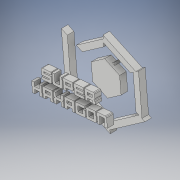
# Autodesk Inventor part: Super-Haxagon
Saved by Autodesk Inventor 2017 (Build 210142000, 142)
## iProperties
Created: 2016-12-10
Part Number: Super-Haxagon
Material: Generic
Document SubType Name: Modeling
Designer: AJ
Density: 1 g/cm^3
Appearance: Default
Author: AJ
Autodesk Inventor part; units mm, degrees
ref_plane "YZ Plane" through (0, 0, 0) normal (1, 0, 0) x (0, 1, 0)
ref_plane "XZ Plane" through (0, 0, 0) normal (0, 1, 0) x (-1, 0, 0)
sketch "Shapes" plane through (0, 0, 0) normal (0, 0, 1) x (1, 0, 0)
  circle A0 centre (0, 0) radius 63.5 construction
  line L0 (52.0162, 36.4221) -> (-5.5344, 63.2584)
  line L1 (-5.5344, 63.2584) -> (-57.5505, 26.8363)
  line L2 (-57.5505, 26.8363) -> (-52.0162, -36.4221)
  line L3 (52.0162, 36.4221) -> (57.5505, -26.8363)
  line L4 (57.5505, -26.8363) -> (5.5344, -63.2584)
  line L5 (5.5344, -63.2584) -> (-52.0162, -36.4221)
  line L6 (0, 0) -> (52.0162, 36.4221) construction
  line L7 (0, 0) -> (63.5, 0) construction
  line L8 (23.2409, 49.8402) -> (26.8363, 57.5505) construction
  line L9 (26.8363, 57.5505) -> (28.9832, 62.1546) construction
  line L10 (28.9832, 62.1546) -> (24.3791, 64.3015)
  line L11 (24.3791, 64.3015) -> (33.277, 71.3627)
  line L12 (33.277, 71.3627) -> (33.5872, 60.0077)
  line L13 (33.5872, 60.0077) -> (28.9832, 62.1546)
  line L14 (28.9832, 62.1546) -> (33.277, 71.3627) construction
  line L15 (0, 0) -> (-57.5505, 26.8363) construction
  line L16 (0, 0) -> (-52.0162, -36.4221) construction
  line L17 (0, 0) -> (5.5344, -63.2584) construction
  line L18 (0, 0) -> (57.5505, -26.8363) construction
  line L19 (0, 0) -> (-5.5344, 63.2584) construction
  line L20 (52.0162, 36.4221) -> (83.2258, 58.2754) construction
  line L21 (57.5505, -26.8363) -> (92.0809, -42.938) construction
  line L22 (5.5344, -63.2584) -> (8.855, -101.2134) construction
  line L23 (-52.0162, -36.4221) -> (-83.2258, -58.2754) construction
  line L24 (-57.5505, 26.8363) -> (-92.0809, 42.938) construction
  line L25 (-9.9619, 113.8651) -> (93.6291, 65.5598)
  line L26 (114.4355, 80.1286) -> (-12.1757, 139.1684)
  line L27 (104.0323, 72.8442) -> (115.1011, -53.6725)
  line L28 (124.8388, 87.413) -> (138.1213, -64.407)
  line L29 (126.6112, -59.0398) -> (12.1757, -139.1684)
  line L30 (149.6314, -69.7743) -> (14.3894, -164.4717)
  line L31 (13.2825, -151.8201) -> (-124.8388, -87.413)
  line L32 (15.4963, -177.1234) -> (-145.6452, -101.9819)
  line L33 (-135.242, -94.6975) -> (-149.6314, 69.7743)
  line L34 (-172.6516, 80.5088) -> (-156.0485, -109.2663)
  line L35 (-92.0809, 42.938) -> (-8.855, 101.2134)
  line L36 (-11.0688, 126.5167) -> (-115.1011, 53.6725)
  line L37 (93.6291, 65.5598) -> (114.4355, 80.1286)
  line L38 (104.0323, 72.8442) -> (124.8388, 87.413)
  line L39 (115.1011, -53.6725) -> (138.1213, -64.407)
  line L40 (126.6112, -59.0398) -> (149.6314, -69.7743)
  line L41 (12.1757, -139.1684) -> (14.3894, -164.4717)
  line L42 (13.2825, -151.8201) -> (15.4963, -177.1234)
  line L43 (-156.0485, -109.2663) -> (-135.242, -94.6975)
  line L44 (-145.6452, -101.9819) -> (-124.8388, -87.413)
  line L45 (-92.0809, 42.938) -> (-115.1011, 53.6725)
  line L46 (-8.855, 101.2134) -> (-11.0688, 126.5167)
  line L47 (-172.6516, 80.5088) -> (-149.6314, 69.7743)
  line L48 (-5.5344, 63.2584) -> (-8.855, 101.2134) construction
  line L49 (-9.9619, 113.8651) -> (-12.1757, 139.1684)
  line L50 (-8.855, 101.2134) -> (-9.9619, 113.8651)
  line L51 (93.6291, 65.5598) -> (104.0323, 72.8442)
  line L52 (115.1011, -53.6725) -> (126.6112, -59.0398)
  line L53 (-124.8388, -87.413) -> (-135.242, -94.6975)
  line L54 (12.1757, -139.1684) -> (13.2825, -151.8201)
  dimension "d0" = 127
  dimension "d1" = 35
  dimension "d2" = 5.08
  dimension "d3" = 10.16
  dimension "d4" = 5.08
  dimension "d28" = 38.1
  dimension "d29" = 25.4
  dimension "d30" = 12.7
  dimension "d31" = 12.7
  dimension "d32" = 12.7
  dimension "d33" = 12.7
  dimension "d34" = 12.7
  constraints: 110 end point, 21 collinear, 19 point on line, 16 equal length, 13 parallel, 3 perpendicular, 1 coincident, 1 horizontal, 1 midpoint, 12 other
  measures "d1" angle of L6 L7
  measures "d2" distance of L8.end L9.end
  measures "d3" distance of L9.end L11.end
  measures "d4" distance of L9.end L10.end
  measures "d28" distance of L0.end L48.end
  measures "d29" distance of L35.end L36.start
  measures "d30" distance of L48.end L25.start
  measures "d31" distance of L25.end L27.start
  measures "d32" distance of L27.end L29.start
  measures "d33" distance of L29.end L31.start
  measures "d34" distance of L31.end L33.start
extrude "Hexagon" add sketch "Shapes" along normal blind 25.4
sketch "Lift" plane through (124.8388, 87.413, 25.4) normal (0.9962, 0.0872, 0) x (0, 0, -1)
  line L0 (25.4, 0) -> (0, 0) projected
  line L1 (0, 0) -> (-101.6, 0)
  dimension "d39" = 101.6
  constraints: 2 end point, 1 horizontal
  measures "d39" distance of L0.end L1.end
ref_plane "Offset Face" through (124.8388, 87.413, 127) normal (0, 0, 1) x (1, 0, 0)
sketch "Words" plane through (124.8388, 87.413, 127) normal (0, 0, 1) x (1, 0, 0)
  line L0 (-308.6212, -54.5376) -> (20.3223, -25.7588) construction
  line L1 (20.3223, -25.7588) -> (28.8231, -122.9237) construction
  line L2 (28.8231, -122.9237) -> (-300.1204, -151.7025) construction
  line L3 (-300.1204, -151.7025) -> (-308.6212, -54.5376) construction
  line L4 (-300.1204, -151.7025) -> (-284.9384, -150.3742)
  line L5 (28.8231, -122.9237) -> (10.8917, -124.4925)
  line L6 (-297.4904, -6.9043) -> (-280.8872, -196.6794) projected
  line L7 (13.2825, -151.8201) -> (0, 0) projected
  line L8 (-72.8226, -50.9909) -> (-130.3732, -24.1547) projected
  line L9 (-129.0892, -38.8306) -> (-130.3732, -24.1547)
  line L10 (-176.8549, -123.8352) -> (-119.3044, -150.6714) projected
  line L11 (-120.5884, -135.9955) -> (-119.3044, -150.6714)
  line L12 (-245.3905, -87.2512) -> (-246.2217, -77.7509)
  line L13 (-246.2217, -77.7509) -> (-217.7439, -75.2594)
  line L14 (-217.7439, -75.2594) -> (-218.1574, -70.5324)
  line L15 (-218.1574, -70.5324) -> (-246.6353, -73.0239)
  line L16 (-246.6353, -73.0239) -> (-248.2956, -54.0464)
  spline S0 degree 2 poles (-248.2956, -54.0464) (-248.4679, -52.0768) (-247.2204, -50.5901) knots 0 0 0 1 1 1
  spline S1 degree 2 poles (-247.2204, -50.5901) (-245.9306, -49.0529) (-243.961, -48.8806) knots 0 0 0 1 1 1
  line L17 (-243.961, -48.8806) -> (-210.7561, -45.9756)
  line L18 (-210.7561, -45.9756) -> (-209.927, -55.4527)
  line L19 (-209.927, -55.4527) -> (-238.3817, -57.9422)
  line L20 (-238.3817, -57.9422) -> (-237.9661, -62.6924)
  line L21 (-237.9661, -62.6924) -> (-209.5114, -60.2029)
  line L22 (-209.5114, -60.2029) -> (-207.8511, -79.1804)
  spline S2 degree 2 poles (-207.8511, -79.1804) (-207.6747, -81.1963) (-208.9686, -82.6871) knots 0 0 0 1 1 1
  spline S3 degree 2 poles (-208.9686, -82.6871) (-210.2624, -84.1779) (-212.1857, -84.3462) knots 0 0 0 1 1 1
  line L23 (-212.1857, -84.3462) -> (-245.3905, -87.2512)
  spline S4 degree 2 poles (-198.8157, -83.1764) (-200.8316, -83.3528) (-202.3183, -82.1053) knots 0 0 0 1 1 1
  spline S5 degree 2 poles (-202.3183, -82.1053) (-203.8091, -80.8114) (-203.9815, -78.8419) knots 0 0 0 1 1 1
  line L24 (-203.9815, -78.8419) -> (-206.8865, -45.637)
  line L25 (-206.8865, -45.637) -> (-197.3862, -44.8058)
  line L26 (-197.3862, -44.8058) -> (-194.8967, -73.2605)
  line L27 (-194.8967, -73.2605) -> (-175.9192, -71.6002)
  line L28 (-175.9192, -71.6002) -> (-178.4086, -43.1455)
  line L29 (-178.4086, -43.1455) -> (-168.9315, -42.3164)
  line L30 (-168.9315, -42.3164) -> (-165.6108, -80.2714)
  line L31 (-165.6108, -80.2714) -> (-198.8157, -83.1764)
  line L32 (-161.7412, -79.9328) -> (-165.0618, -41.9778)
  line L33 (-165.0618, -41.9778) -> (-127.1068, -38.6572)
  line L34 (-127.1068, -38.6572) -> (-125.0309, -62.3849)
  spline S6 degree 2 poles (-125.0309, -62.3849) (-124.8566, -64.3776) (-126.1504, -65.8684) knots 0 0 0 1 1 1
  spline S7 degree 2 poles (-126.1504, -65.8684) (-127.4443, -67.3592) (-129.3675, -67.5275) knots 0 0 0 1 1 1
  line L35 (-129.3675, -67.5275) -> (-153.072, -69.6013)
  line L36 (-153.072, -69.6013) -> (-152.2409, -79.1017)
  line L37 (-152.2409, -79.1017) -> (-161.7412, -79.9328)
  line L38 (-134.9237, -58.4638) -> (-135.7548, -48.9635)
  line L39 (-135.7548, -48.9635) -> (-154.7323, -50.6238)
  line L40 (-154.7323, -50.6238) -> (-153.9012, -60.1242)
  line L41 (-153.9012, -60.1242) -> (-134.9237, -58.4638)
  spline S8 degree 2 poles (-115.1664, -75.8581) (-117.1823, -76.0344) (-118.669, -74.7869) knots 0 0 0 1 1 1
  spline S9 degree 2 poles (-118.669, -74.7869) (-120.1598, -73.4931) (-120.3321, -71.5235) knots 0 0 0 1 1 1
  line L42 (-120.3321, -71.5235) -> (-123.2372, -38.3186)
  line L43 (-123.2372, -38.3186) -> (-85.2821, -34.998)
  line L44 (-85.2821, -34.998) -> (-84.453, -44.4752)
  line L45 (-84.453, -44.4752) -> (-112.9077, -46.9646)
  line L46 (-112.9077, -46.9646) -> (-112.4921, -51.7148)
  line L47 (-112.4921, -51.7148) -> (-84.0374, -49.2253)
  line L48 (-84.0374, -49.2253) -> (-83.2062, -58.7257)
  line L49 (-83.2062, -58.7257) -> (-111.6609, -61.2151)
  line L50 (-111.6609, -61.2151) -> (-111.2474, -65.9421)
  line L51 (-111.2474, -65.9421) -> (-82.7927, -63.4527)
  line L52 (-82.7927, -63.4527) -> (-81.9615, -72.953)
  line L53 (-81.9615, -72.953) -> (-115.1664, -75.8581)
  line L54 (-78.0919, -72.6145) -> (-81.4125, -34.6595)
  line L55 (-81.4125, -34.6595) -> (-48.2076, -31.7544)
  spline S10 degree 2 poles (-48.2076, -31.7544) (-46.2381, -31.5821) (-44.7473, -32.8759) knots 0 0 0 1 1 1
  spline S11 degree 2 poles (-44.7473, -32.8759) (-43.2102, -34.1658) (-43.0419, -36.089) knots 0 0 0 1 1 1
  line L56 (-43.0419, -36.089) -> (-41.7972, -50.3163)
  spline S12 degree 2 poles (-41.7972, -50.3163) (-41.6228, -52.3091) (-42.9146, -53.823) knots 0 0 0 1 1 1
  spline S13 degree 2 poles (-42.9146, -53.823) (-44.2085, -55.3138) (-46.1317, -55.4821) knots 0 0 0 1 1 1
  spline S14 degree 2 poles (-46.1317, -55.4821) (-44.1622, -55.3098) (-42.6714, -56.6036) knots 0 0 0 1 1 1
  spline S15 degree 2 poles (-42.6714, -56.6036) (-41.1363, -57.8703) (-40.968, -59.7935) knots 0 0 0 1 1 1
  line L57 (-40.968, -59.7935) -> (-40.1368, -69.2938)
  line L58 (-40.1368, -69.2938) -> (-49.614, -70.123)
  line L59 (-49.614, -70.123) -> (-50.4452, -60.6226)
  line L60 (-50.4452, -60.6226) -> (-69.4227, -62.283)
  line L61 (-69.4227, -62.283) -> (-68.5915, -71.7833)
  line L62 (-68.5915, -71.7833) -> (-78.0919, -72.6145)
  line L63 (-51.2743, -51.1455) -> (-52.1055, -41.6451)
  line L64 (-52.1055, -41.6451) -> (-71.083, -43.3055)
  line L65 (-71.083, -43.3055) -> (-70.2518, -52.8058)
  line L66 (-70.2518, -52.8058) -> (-51.2743, -51.1455)
  line L67 (-282.0424, -150.036) -> (-285.363, -112.081)
  line L68 (-285.363, -112.081) -> (-275.8627, -111.2498)
  line L69 (-275.8627, -111.2498) -> (-274.6179, -125.4771)
  line L70 (-274.6179, -125.4771) -> (-255.6404, -123.8168)
  line L71 (-255.6404, -123.8168) -> (-256.8852, -109.5895)
  line L72 (-256.8852, -109.5895) -> (-247.408, -108.7603)
  line L73 (-247.408, -108.7603) -> (-244.0874, -146.7154)
  line L74 (-244.0874, -146.7154) -> (-253.5645, -147.5445)
  line L75 (-253.5645, -147.5445) -> (-254.8093, -133.3172)
  line L76 (-254.8093, -133.3172) -> (-273.7868, -134.9775)
  line L77 (-273.7868, -134.9775) -> (-272.542, -149.2048)
  line L78 (-272.542, -149.2048) -> (-282.0424, -150.036)
  line L79 (-240.2177, -146.3768) -> (-243.1228, -113.172)
  spline S16 degree 2 poles (-243.1228, -113.172) (-243.2951, -111.2024) (-242.0476, -109.7157) knots 0 0 0 1 1 1
  spline S17 degree 2 poles (-242.0476, -109.7157) (-240.7578, -108.1785) (-238.7882, -108.0062) knots 0 0 0 1 1 1
  line L80 (-238.7882, -108.0062) -> (-205.5833, -105.1012)
  line L81 (-205.5833, -105.1012) -> (-202.2627, -143.0562)
  line L82 (-202.2627, -143.0562) -> (-211.7399, -143.8853)
  line L83 (-211.7399, -143.8853) -> (-212.571, -134.385)
  line L84 (-212.571, -134.385) -> (-231.5485, -136.0453)
  line L85 (-231.5485, -136.0453) -> (-230.7174, -145.5456)
  line L86 (-230.7174, -145.5456) -> (-240.2177, -146.3768)
  line L87 (-213.4002, -124.9078) -> (-214.2313, -115.4075)
  line L88 (-214.2313, -115.4075) -> (-233.2089, -117.0678)
  line L89 (-233.2089, -117.0678) -> (-232.3777, -126.5681)
  line L90 (-232.3777, -126.5681) -> (-213.4002, -124.9078)
  line L91 (-198.393, -142.7176) -> (-199.6378, -128.4903)
  spline S18 degree 2 poles (-199.6378, -128.4903) (-199.8101, -126.5207) (-198.5626, -125.034) knots 0 0 0 1 1 1
  spline S19 degree 2 poles (-198.5626, -125.034) (-197.2728, -123.4969) (-195.3032, -123.3245) knots 0 0 0 1 1 1
  spline S20 degree 2 poles (-195.3032, -123.3245) (-197.3191, -123.5009) (-198.8058, -122.2534) knots 0 0 0 1 1 1
  spline S21 degree 2 poles (-198.8058, -122.2534) (-200.2966, -120.9595) (-200.4689, -118.99) knots 0 0 0 1 1 1
  line L92 (-200.4689, -118.99) -> (-201.7137, -104.7626)
  line L93 (-201.7137, -104.7626) -> (-192.2133, -103.9314)
  line L94 (-192.2133, -103.9314) -> (-190.9686, -118.1588)
  line L95 (-190.9686, -118.1588) -> (-171.9911, -116.4985)
  line L96 (-171.9911, -116.4985) -> (-173.2358, -102.2711)
  line L97 (-173.2358, -102.2711) -> (-163.7587, -101.442)
  line L98 (-163.7587, -101.442) -> (-162.5139, -115.6693)
  spline S22 degree 2 poles (-162.5139, -115.6693) (-162.3376, -117.6852) (-163.6314, -119.176) knots 0 0 0 1 1 1
  spline S23 degree 2 poles (-163.6314, -119.176) (-164.9253, -120.6668) (-166.8485, -120.8351) knots 0 0 0 1 1 1
  spline S24 degree 2 poles (-166.8485, -120.8351) (-164.8789, -120.6628) (-163.3881, -121.9566) knots 0 0 0 1 1 1
  spline S25 degree 2 poles (-163.3881, -121.9566) (-161.851, -123.2464) (-161.6828, -125.1697) knots 0 0 0 1 1 1
  line L99 (-161.6828, -125.1697) -> (-160.438, -139.397)
  line L100 (-160.438, -139.397) -> (-169.9152, -140.2261)
  line L101 (-169.9152, -140.2261) -> (-171.1599, -125.9988)
  line L102 (-171.1599, -125.9988) -> (-190.1374, -127.6591)
  line L103 (-190.1374, -127.6591) -> (-188.8927, -141.8865)
  line L104 (-188.8927, -141.8865) -> (-198.393, -142.7176)
  line L105 (-156.5684, -139.0584) -> (-159.4734, -105.8536)
  spline S26 degree 2 poles (-159.4734, -105.8536) (-159.6457, -103.884) (-158.3982, -102.3973) knots 0 0 0 1 1 1
  spline S27 degree 2 poles (-158.3982, -102.3973) (-157.1084, -100.8602) (-155.1388, -100.6878) knots 0 0 0 1 1 1
  line L106 (-155.1388, -100.6878) -> (-121.934, -97.7828)
  line L107 (-121.934, -97.7828) -> (-118.6134, -135.7378)
  line L108 (-118.6134, -135.7378) -> (-128.0905, -136.567)
  line L109 (-128.0905, -136.567) -> (-128.9217, -127.0666)
  line L110 (-128.9217, -127.0666) -> (-147.8992, -128.7269)
  line L111 (-147.8992, -128.7269) -> (-147.068, -138.2273)
  line L112 (-147.068, -138.2273) -> (-156.5684, -139.0584)
  line L113 (-129.7508, -117.5894) -> (-130.582, -108.0891)
  line L114 (-130.582, -108.0891) -> (-149.5595, -109.7494)
  line L115 (-149.5595, -109.7494) -> (-148.7283, -119.2498)
  line L116 (-148.7283, -119.2498) -> (-129.7508, -117.5894)
  line L117 (-114.7437, -135.3993) -> (-118.0643, -97.4442)
  line L118 (-118.0643, -97.4442) -> (-80.1093, -94.1236)
  line L119 (-80.1093, -94.1236) -> (-79.2802, -103.6008)
  line L120 (-79.2802, -103.6008) -> (-107.7348, -106.0902)
  line L121 (-107.7348, -106.0902) -> (-106.0745, -125.0677)
  line L122 (-106.0745, -125.0677) -> (-87.097, -123.4074)
  line L123 (-87.097, -123.4074) -> (-88.3418, -109.1801)
  line L124 (-88.3418, -109.1801) -> (-78.8646, -108.3509)
  line L125 (-78.8646, -108.3509) -> (-77.2043, -127.3285)
  spline S28 degree 2 poles (-77.2043, -127.3285) (-77.0279, -129.3444) (-78.3218, -130.8352) knots 0 0 0 1 1 1
  spline S29 degree 2 poles (-78.3218, -130.8352) (-79.6156, -132.326) (-81.5389, -132.4942) knots 0 0 0 1 1 1
  line L126 (-81.5389, -132.4942) -> (-114.7437, -135.3993)
  line L127 (-72.919, -131.7401) -> (-75.8241, -98.5352)
  spline S30 degree 2 poles (-75.8241, -98.5352) (-75.9964, -96.5656) (-74.7489, -95.0789) knots 0 0 0 1 1 1
  spline S31 degree 2 poles (-74.7489, -95.0789) (-73.4591, -93.5418) (-71.4895, -93.3695) knots 0 0 0 1 1 1
  line L128 (-71.4895, -93.3695) -> (-38.2846, -90.4644)
  line L129 (-38.2846, -90.4644) -> (-35.3796, -123.6693)
  spline S32 degree 2 poles (-35.3796, -123.6693) (-35.2032, -125.6852) (-36.4971, -127.176) knots 0 0 0 1 1 1
  spline S33 degree 2 poles (-36.4971, -127.176) (-37.7909, -128.6668) (-39.7142, -128.835) knots 0 0 0 1 1 1
  line L130 (-39.7142, -128.835) -> (-72.919, -131.7401)
  line L131 (-45.2724, -119.7482) -> (-46.9327, -100.7707)
  line L132 (-46.9327, -100.7707) -> (-65.9102, -102.4311)
  line L133 (-65.9102, -102.4311) -> (-64.2499, -121.4086)
  line L134 (-64.2499, -121.4086) -> (-45.2724, -119.7482)
  line L135 (-31.0944, -128.0809) -> (-34.415, -90.1259)
  line L136 (-34.415, -90.1259) -> (-1.2102, -87.2208)
  spline S34 degree 2 poles (-1.2102, -87.2208) (0.7594, -87.0485) (2.2502, -88.3424) knots 0 0 0 1 1 1
  spline S35 degree 2 poles (2.2502, -88.3424) (3.7873, -89.6322) (3.9556, -91.5554) knots 0 0 0 1 1 1
  line L137 (3.9556, -91.5554) -> (6.8607, -124.7603)
  line L138 (6.8607, -124.7603) -> (-2.6165, -125.5894)
  line L139 (-2.6165, -125.5894) -> (-5.108, -97.1116)
  line L140 (-5.108, -97.1116) -> (-24.0855, -98.7719)
  line L141 (-24.0855, -98.7719) -> (-21.594, -127.2497)
  line L142 (-21.594, -127.2497) -> (-31.0944, -128.0809)
  dimension "d42" = 330.2
  dimension "d43" = 97.536
  dimension "d44" = 15.24
  constraints: 8 end point, 6 point on line, 2 perpendicular, 1 coincident, 1 collinear, 1 parallel, 2 other
  measures "d42" distance of L0.start L0.end
  measures "d43" distance of L2.end L0.start
  measures "d44" distance of L2.end L4.end
extrude "Text" add sketch "Words" along normal blind 25.4 contours L33 L34 S6 S7 L35 L36 L37 L32 | L45 L46 L47 L48 L49 L50 L51 L52 L53 S8 S9 L42 L43 L8 | L8 L43 L44 L45 | L54 L55 S10 S11 L56 S12 S13 S14 S15 L57 L58 L59 L60 L61 L62 | L102 L103 L104 L91 S18 S19 S20 S21 L92 L93 L94 L95 L96 L97 L98 S22 S23 S24 S25 L99 L10 L101 | L105 S26 S27 L106 L107 L108 L109 L110 L111 L10 | L10 L111 L112 L105 | L10 L99 L100 L101 | L12 L13 L14 L15 L16 S0 S1 L17 L18 L19 L20 L21 L22 S2 S3 L23 | S4 S5 L24 L25 L26 L27 L28 L29 L30 L31 | L67 L68 L69 L70 L71 L72 L73 L74 L75 L76 L77 L78 | L79 S16 S17 L80 L81 L82 L83 L84 L85 L86 | L117 L118 L119 L120 L121 L122 L123 L124 L125 S28 S29 L126 | L127 S30 S31 L128 L129 S32 S33 L130 | L135 L136 S34 S35 L137 L138 L139 L140 L141 L142
body "Solid2"
